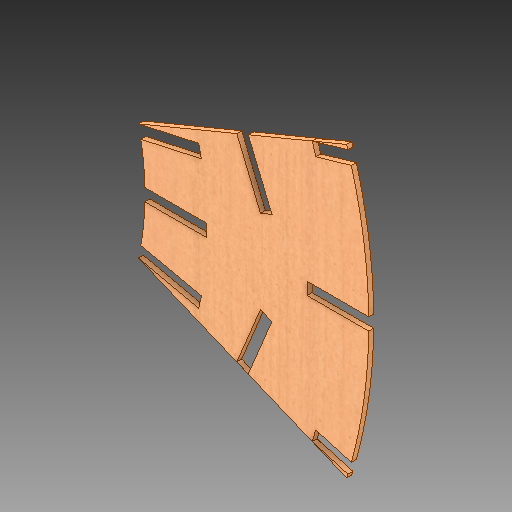
# Autodesk Inventor part: internalSupportTop1
Saved by Autodesk Inventor 2019 (Build 230136000, 136)
## iProperties
Company: FABLAB Torino
Created: 2019-01-11
Part Number: internalSupportTop1
Material: Wood (Cherry)
Document SubType Name: Modeling
Designer: Giancarlo
Density: 0.63 g/cm^3
Appearance: Cherry - Natural Low Gloss
Mass: 49.9686 g
Surface Area: 569.703 cm^2
Volume: 79.3152 cm^3
Description: MultiLayer 10mm
Author: Giancarlo
Title: La Panca - Flower Vase
Subject: Construction MOld
Autodesk Inventor part; units mm, degrees
ref_plane "YZ Plane" through (0, 0, 0) normal (1, 0, 0) x (0, 1, 0)
ref_plane "XZ Plane" through (0, 0, 0) normal (0, 1, 0) x (-1, 0, 0)
ref_plane "Work Plane1" through (0, 0, 0) normal (0, 0, 1) x (1, 0, 0)
sketch "Sketch2" plane through (0, 0, 0) normal (0, 0, 1) x (1, 0, 0)
  spline S0 degree 3 poles (62.9391, 116.7394) (68.6793, 98.401) (73.0646, 79.638) (79.1979, 40.5999) (80.7828, 20.2998) (80.7828, 0) (80.7828, -20.2998) (79.1979, -40.5999) (73.0646, -79.638) (68.6793, -98.401) (62.9391, -116.7394) knots -24.034595 -24.034595 -24.034595 -24.034595 -18.269852 -18.269852 -12.179902 -12.179902 -12.179902 -6.089951 -6.089951 -0.325208 -0.325208 -0.325208 -0.325208 projected
  spline S1 degree 3 poles (-105.4906, -46.9736) (-103.8187, -39.6955) (-102.5357, -32.328) (-100.6605, -16.6479) (-100.1646, -8.324) (-100.1646, 0) (-100.1646, 8.324) (-100.6605, 16.6479) (-102.5357, 32.328) (-103.8187, 39.6955) (-105.4906, 46.9736) knots -9.731856 -9.731856 -9.731856 -9.731856 -7.491562 -7.491562 -4.994375 -4.994375 -4.994375 -2.497187 -2.497187 -0.256894 -0.256894 -0.256894 -0.256894 projected
  line L0 (62.9391, -116.7394) -> (-105.4906, -46.9736)
  line L1 (-105.4906, 46.9736) -> (62.9391, 116.7394)
  point P0 (0, 0)
  constraints: 4 end point
extrude "Extrusion2" add sketch "Sketch2" along normal blind 4
sketch "Sketch3" plane through (0, 0, 0) normal (0, 0, -1) x (-1, 0, 0)
  line L0 (50.2161, -5) -> (50.2161, 5)
  line L1 (50.2161, 5) -> (101.2252, 5)
  line L2 (101.2252, 5) -> (101.2252, -5)
  line L3 (101.2252, -5) -> (50.2161, -5)
  line L4 (56.6852, -57.7449) -> (54.5301, -47.9799)
  line L5 (54.5301, -47.9799) -> (104.3389, -36.9871)
  line L6 (104.3389, -36.9871) -> (106.4941, -46.7521)
  line L7 (106.4941, -46.7521) -> (56.6852, -57.7449)
  line L8 (-2.4688, -37.5673) -> (6.77, -33.7404)
  line L9 (6.77, -33.7404) -> (25.9042, -79.9344)
  line L10 (25.9042, -79.9344) -> (16.6654, -83.7613)
  line L11 (16.6654, -83.7613) -> (-2.4688, -37.5673)
  line L12 (6.761, 33.7491) -> (-2.4778, 37.576)
  line L13 (-2.4778, 37.576) -> (16.6564, 83.7699)
  line L14 (16.6564, 83.7699) -> (25.8952, 79.9431)
  line L15 (25.8952, 79.9431) -> (6.761, 33.7491)
  line L16 (-30.9132, 5.0001) -> (-30.9132, -4.9999)
  line L17 (-30.9132, -4.9999) -> (-81.9207, -4.9999)
  line L18 (-81.9207, -4.9999) -> (-81.9207, 5.0001)
  line L19 (-81.9207, 5.0001) -> (-30.9132, 5.0001)
  line L20 (0, 0) -> (-130.3795, 0) construction
  line L21 (56.6852, 57.7449) -> (54.5301, 47.9799)
  line L22 (54.5301, 47.9799) -> (104.3389, 36.9871)
  line L23 (104.3389, 36.9871) -> (106.4941, 46.7521)
  line L24 (106.4941, 46.7521) -> (56.6852, 57.7449)
  constraints: 50 end point, 5 horizontal, 4 symmetric about line, 4 vertical, 32 other
extrude "Extrusion3" cut sketch "Sketch3" against normal through all
sketch "Sketch4" plane through (0, 0, 0) normal (0, 0, -1) x (-1, 0, 0)
  line L0 (-63.9494, -113.5716) -> (-35.1346, -105.2224)
  line L1 (-35.1346, -105.2224) -> (-37.9176, -95.6175)
  line L2 (-37.9176, -95.6175) -> (-66.7324, -103.9667)
  line L3 (-66.7324, -103.9667) -> (-63.9494, -113.5716)
  line L4 (-62.9391, -116.7394) -> (105.4906, -46.9736) construction
  line L5 (0, 0) -> (-102.4259, 0) construction
  line L6 (-63.9494, 113.5716) -> (-35.1346, 105.2224)
  line L7 (-35.1346, 105.2224) -> (-37.9176, 95.6175)
  line L8 (-37.9176, 95.6175) -> (-66.7324, 103.9667)
  line L9 (-66.7324, 103.9667) -> (-63.9494, 113.5716)
  point P0 (-80.7508, -4.9999)
  point P1 (-65.3409, -108.7691)
  point P2 (-62.9391, 116.7394)
  point P3 (-65.3409, 108.7691)
  dimension "d21" = 30
  dimension "d22" = 10
  constraints: 18 end point, 6 symmetric about line, 2 parallel, 1 horizontal, 1 midpoint, 1 perpendicular, 1 point on line, 3 other
  measures "d21" distance of L2.end L1.end
  measures "d22" distance of L1.end L0.end
extrude "Extrusion4" cut sketch "Sketch4" against normal through all
body "Solid2"
